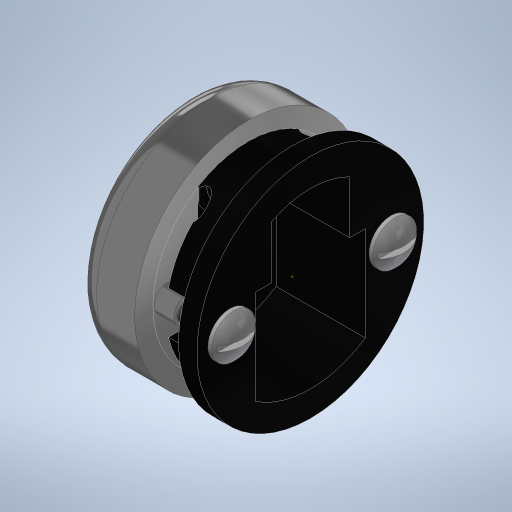
# Autodesk Inventor part: Cup glass T6
Saved by Autodesk Inventor 2024 (Build 280153000, 153)
## iProperties
Created: 2014-01-02
Part Number: Cup glass T6
Material: Generic
Document SubType Name: Modeling
Designer: G. Kazokaitis
Density: 1 g/cm^3
Appearance: Default
Author: G. Kazokaitis
Autodesk Inventor part; units mm, degrees
ref_plane "YZ Plane" through (0, 0, 0) normal (1, 0, 0) x (0, 1, 0)
ref_plane "XZ Plane" through (0, 0, 0) normal (0, 1, 0) x (-1, 0, 0)
sketch "Sketch1" plane through (0, 0, 0) normal (0, 0, 1) x (1, 0, 0)
  line L0 (0, 0) -> (8.2, 0)
  line L1 (0, 0) -> (0, -12.5)
  line L2 (3, -15.5) -> (8.2, -15.5)
  line L3 (8.2, -15.5) -> (8.2, 0)
  arc A0 (0, -12.5) -> (3, -15.5) centre (3, -12.5) ccw
  dimension "d0" = 8.2
  dimension "d1" = 3
  dimension "d2" = 31
  constraints: 8 end point, 2 perpendicular, 2 point on circle, 2 tangent, 1 centre point, 1 horizontal, 1 parallel
  measures "d0" distance of L0.start L0.end
  measures "d1" radius of A0
  measures "d2" diameter of L2 L0
revolve "Revolution1" add sketch "Sketch1" angle 360 about axis through (0, 0, 0) along (1, 0, 0)
sketch "Sketch2" plane through (8.2, 0, 0) normal (1, 0, 0) x (0, 0, -1)
  line L0 (-4.6944, -9) -> (9.3808, -9)
  arc A0 (9.3808, -9) -> (13, 0) centre (0, 0) ccw
  arc A1 (13, 0) -> (9.3808, 9) centre (0, 0) ccw
  line L1 (9.3808, 9) -> (-4.7386, 9)
  line L2 (-4.7386, 9) -> (-4.7386, 7)
  line L3 (-4.7386, 7) -> (-10.9545, 7)
  arc A2 (-10.9545, 7) -> (-11.1405, -6.7) centre (0, 0) ccw
  line L4 (-11.1405, -6.7) -> (-4.6944, -6.7)
  line L5 (-4.6944, -6.7) -> (-4.6944, -9)
  circle A3 centre (0, 0) radius 15.5
  constraints: 12 end point, 6 point on circle, 4 centre point, 4 horizontal, 2 vertical, 15 other
extrude "Extrusion1" cut sketch "Sketch2" against normal blind 5 contours L5 L4 A2 L3 L2 L1 A1 A0 L0
sketch "Sketch3" plane through (8.2, 0, 0) normal (1, 0, 0) x (0, 0, -1)
  arc A0 (9.3808, -9) -> (9.3808, 9) centre (0, 0) ccw projected
  circle A1 centre (0, 11) radius 1.85
  circle A2 centre (0, -11) radius 1.85
  dimension "d6" = 3.7
  dimension "d7" = 3.7
  dimension "d8" = 11
  dimension "d9" = 11
  constraints: 2 centre point
  measures "d6" diameter of A1
  measures "d7" diameter of A2
  measures "d8" distance of A0.centre A1.centre
  measures "d9" distance of A0.centre A2.centre
extrude "Extrusion2" add sketch "Sketch3" along normal blind 2.7
hole "Hole1" at (10.9, 11, 0) direction (-1, 0, 0) diameter 2.459 depth 8 tip angle 118 thread size "M3x0.5" class "6H" standard "ISO Metric profile"
hole "Hole2" at (10.9, -11, 0) direction (-1, 0, 0) diameter 2.459 depth 8 tip angle 118 thread size "M3x0.5" class "6H" standard "ISO Metric profile"
sketch "Sketch4" plane through (8.2, 0, 0) normal (1, 0, 0) x (0, 0, -1)
  circle A0 centre (0, 0) radius 15.5 projected
  circle A1 centre (0, 0) radius 13
  dimension "d30" = 26
  constraints: 1 centre point, 1 coincident
  measures "d30" diameter of A1
extrude "Extrusion3" add sketch "Sketch4" along normal blind 6 separate body contours A1
sketch "Sketch6" plane through (0, 0, 0) normal (0, 1, 0) x (-1, 0, 0)
  line L0 (-6.2, 0) -> (-16.7, 0)
  line L1 (-3, 0) -> (-3, 13)
  line L2 (-3, 13) -> (-14.2, 13)
  line L3 (-14.2, 13) -> (-14.2, 15.5)
  line L4 (-14.2, 15.5) -> (-16.7, 15.5)
  line L5 (-16.7, 15.5) -> (-16.7, 0)
  line L6 (-8.2, -15.5) -> (-8.2, 15.5) projected
  line L7 (-3, 0) -> (-6.2, 0)
  point P0 (0, 0)
  dimension "d33" = 26
  dimension "d34" = 31
  dimension "d35" = 2.5
  dimension "d59" = 11.2
  dimension "d60" = 6
  constraints: 14 end point, 3 parallel, 3 perpendicular, 2 point on line, 1 horizontal
  measures "d33" diameter of L2 L0
  measures "d34" diameter of L4 L0
  measures "d35" distance of L3.end L4.end
  measures "d59" distance between parallel lines of L3 L1
  measures "d60" distance between parallel lines of L6 L3
revolve "Revolution2" add sketch "Sketch6" angle 360 about axis through (6.2, 0, 0) along (1, 0, 0) separate body
sketch "Sketch7" plane through (3, 0, 0) normal (-1, 0, 0) x (0, 0, 1)
  line L0 (4.7, 9) -> (4.7, 6.85)
  line L1 (-9.3808, 9) -> (4.7, 9)
  line L2 (4.7, 6.85) -> (11.0489, 6.85)
  arc A0 (11.0489, 6.85) -> (-9.3808, 9) centre (0, 0) ccw
  circle A1 centre (0, 0) radius 13
  constraints: 6 end point, 2 centre point, 2 point on circle, 1 concentric
extrude "Extrusion4" cut sketch "Sketch7" against normal blind 7 contours L1 A0 L2 L0 bodies 3
sketch "Sketch8" plane through (10, 0, 0) normal (-1, 0, 0) x (0, 0, 1)
  line L0 (-2.9, 12.6724) -> (-2.9, 9)
  line L1 (2.9, 9) -> (2.9, 12.6724)
  line L2 (-9.3808, 9) -> (4.7, 9)
  arc A0 (11.0489, 6.85) -> (-9.3808, 9) centre (0, 0) ccw
  line L3 (-2.9, 9) -> (2.9, 9)
  arc A1 (2.9, 12.6724) -> (-2.9, 12.6724) centre (0, 0) ccw
  line L4 (4.7, 6.85) -> (11.0489, 6.85)
  line L5 (4.7, 9) -> (4.7, 6.85)
  constraints: 12 end point, 4 point on circle, 2 centre point, 1 collinear, 1 concentric
extrude "Extrusion5" cut sketch "Sketch8" against normal blind 3.2 contours A0 L1 L2 L0 bodies 3
sketch "Sketch9" plane through (13.2, 0, 0) normal (-1, 0, 0) x (0, 0, 1)
  arc A0 (2.9, 12.6724) -> (-2.9, 12.6724) centre (0, 0) ccw projected
  point P0 (0, 11)
  dimension "d42" = 11
  measures "d42" distance of point (0, 11) A0.centre
hole "Hole3" at (13.2, 11, 0) direction (1, 0, 0) diameter 3.1 end through all bodies 3
mirror "Mirror1" about plane through (0, 0, 0) normal (0, 1, 0) of "Hole3", "Extrusion5", "Extrusion4" bodies 3
sketch "Sketch10" plane through (16.7, 0, 0) normal (1, 0, 0) x (0, 0, -1)
  line L0 (-4.7, 6.85) -> (-11.0489, 6.85)
  line L1 (-4.7, 9) -> (-4.7, 6.85)
  line L2 (-2.9, 9) -> (-4.7, 9)
  line L3 (2.9, 9) -> (-2.9, 9)
  line L4 (9.3808, 9) -> (2.9, 9)
  line L5 (9.3808, -9) -> (2.9, -9)
  line L6 (2.9, -9) -> (-2.9, -9)
  line L7 (-2.9, -9) -> (-4.7, -9)
  line L8 (-4.7, -9) -> (-4.7, -6.85)
  line L9 (-4.7, -6.85) -> (-11.0489, -6.85)
  line L10 (-10.4052, 5.35) -> (-3.2, 5.35)
  line L11 (-3.2, 5.35) -> (-3.2, 7.5)
  line L12 (-3.2, 7.5) -> (-2.9, 7.5)
  line L13 (-2.9, 7.5) -> (2.9, 7.5)
  line L14 (2.9, 7.5) -> (9.725, 7.5)
  line L15 (-10.4052, -5.35) -> (-3.2, -5.35)
  line L16 (-3.2, -5.35) -> (-3.2, -7.5)
  line L17 (-3.2, -7.5) -> (-2.9, -7.5)
  line L18 (-2.9, -7.5) -> (2.9, -7.5)
  line L19 (2.9, -7.5) -> (9.725, -7.5)
  circle A0 centre (0, 0) radius 13
  arc A1 (-10.4052, 5.35) -> (-10.4052, -5.35) centre (0, 0) ccw
  arc A2 (9.725, -7.5) -> (9.725, 7.5) centre (-1.5, 0) ccw
  circle A3 centre (0, -11) radius 1.55
  circle A4 centre (0, 11) radius 1.55
  dimension "d50" = 1.5
  dimension "d51" = 1.5
  dimension "d52" = 1.5
  dimension "d53" = 1.5
  dimension "d54" = 11.7
  dimension "d55" = 1.5
  dimension "d56" = 13.5
  constraints: 40 end point, 5 centre point, 4 point on circle, 1 vertical alignment, 4 other
  measures "d50" distance between parallel lines of L14 L4
  measures "d51" distance between parallel lines of L5 L19
  measures "d52" distance between parallel lines of L10 L0
  measures "d53" distance between parallel lines of L15 L9
  measures "d54" radius of A1
  measures "d55" distance of A0.centre A2.centre
  measures "d56" radius of A2
extrude "Extrusion6" cut sketch "Sketch10" against normal blind 12.2 contours L10 L11 L12 L13 L14 A2 L19 L18 L17 L16 L15 A1 bodies 3
sketch "Sketch11" plane through (3, 6.85, 11.0489) normal (0, 1, 0) x (1, 0, 0)
  line L0 (0, 0) -> (0, 6.3489) projected
  line L1 (3.7, 4.5) -> (6.2, 4.5) construction
  line L2 (6.2, 4.5) -> (6.2, 1) construction
  line L3 (6.2, 1) -> (3.7, 1) construction
  line L4 (3.7, 1) -> (3.7, 4.5) construction
  point P0 (-3, 11.0489)
  dimension "d61" = 1
  dimension "d62" = 3.7
  dimension "d63" = 3.5
  dimension "d64" = 2.5
  constraints: 8 end point, 2 parallel, 1 horizontal, 1 perpendicular
  measures "d61" distance from line of L0.start L3
  measures "d62" distance between parallel lines of L4 L0
  measures "d63" distance of L3.end L1.start
  measures "d64" distance of L2.end L3.end
hole "Hole4" at (9.2, 6.85, 10.0489) at (6.7, 6.85, 6.5489) direction (0, -1, 0) diameter 2.6 end through all bodies 3
ref_plane "Work Plane1" through (59.1314, 11, 0) normal (0, 1, 0) x (-1, 0, 0)
sketch "Sketch12" plane through (59.1314, 11, 0) normal (0, 1, 0) x (-1, 0, 0)
  line L0 (42.4314, 3) -> (42.4314, 1.5)
  line L1 (42.4314, 1.5) -> (56.4314, 1.5)
  line L2 (56.4314, 1.5) -> (56.4314, 0)
  line L3 (56.4314, 0) -> (40.5771, 0)
  arc A0 (41.9314, 3) -> (40.5771, 0) centre (44.5771, 0) ccw
  line L4 (41.9314, 3) -> (42.4314, 3)
  line L5 (42.4314, 3.2) -> (42.4314, -9.725) projected
  point P0 (59.1314, 0)
  point P1 (42.4314, 0)
  point P2 (42.4314, 2.25)
  point P3 (42.4314, 0)
  dimension "d73" = 3
  dimension "d74" = 14
  dimension "d75" = 6
  dimension "d76" = 0.5
  dimension "d77" = 4
  constraints: 10 end point, 3 parallel, 3 point on line, 2 point on circle, 1 centre point, 1 midpoint, 1 perpendicular, 1 vertical, 1 vertical alignment
  measures "d73" diameter of L1 L3
  measures "d74" distance from line of L2.end L0
  measures "d75" diameter of L4 L3
  measures "d76" distance of L4.start L0.start
  measures "d77" radius of A0
revolve "Revolution3" add sketch "Sketch12" angle 360 about axis through (2.7, 11, 0) along (1, 0, 0) separate body
sketch "Sketch13" plane through (59.1314, 11, 0) normal (0, 1, 0) x (-1, 0, 0)
  line L0 (40.5771, 0.3456) -> (41.5771, 0.3456)
  line L1 (41.5771, 0.3456) -> (41.5771, -0.4544)
  line L2 (41.5771, -0.4544) -> (40.5771, -0.4544)
  line L3 (40.5771, -0.4544) -> (40.5771, 0.3456)
  arc A0 (41.9314, 3) -> (41.9314, -3) centre (44.5771, 0) ccw projected
  point P0 (59.1314, 0)
  dimension "d79" = 0.8
  dimension "d80" = 1
  constraints: 8 end point, 2 parallel, 1 horizontal, 1 perpendicular, 1 tangent
  measures "d79" distance of L2.end L0.start
  measures "d80" distance of L0.start L0.end
extrude "Extrusion7" cut sketch "Sketch13" along normal through all both and the other way through all bodies 4
thread "Thread1" size "M3x0.5" class "6g" standard "ANSI Metric M Profile" full length
mirror "Mirror2" about plane through (0, 0, 0) normal (0, 1, 0) bodies 4
sketch "Sketch15" plane through (14.2, 0, 0) normal (-1, 0, 0) x (0, 0, 1)
  circle A0 centre (0, 0) radius 15.5 projected
  circle A1 centre (0, 0) radius 13 projected
  constraints: 1 coincident
equation "\"d31\" = Glass_thickness"
equation "\"d60\" = Glass_thickness"
equation "\"Glass_thickness\" = 6"
